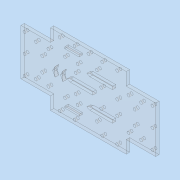
# Autodesk Inventor part: 底盘设计3.0
Saved by Autodesk Inventor 2019 (Build 230136000, 136)
## iProperties
Created: 2020-10-19
Part Number: 底盘设计3.0
Material: 聚碳酸酯，透明
Document SubType Name: Modeling
Designer: Wang Hua
Density: 1.2 g/cm^3
Appearance: 聚碳酸酯 - 透明
Author: Wang Hua
Autodesk Inventor part; units mm, degrees
ref_plane "YZ Plane" through (0, 0, 0) normal (1, 0, 0) x (0, 1, 0)
ref_plane "XZ Plane" through (0, 0, 0) normal (0, 1, 0) x (-1, 0, 0)
ref_plane "XY Plane" through (0, 0, 0) normal (0, 0, 1) x (1, 0, 0)
sketch "草图1" plane through (0, 0, 0) normal (0, 0, 1) x (1, 0, 0)
  line L0 (45, -42.5) -> (-45, -42.5)
  line L1 (-80, -27.5) -> (-80, 27.5)
  line L2 (-45, 42.5) -> (45, 42.5)
  line L3 (80, 27.5) -> (80, -27.5)
  line L4 (80, -42.5) -> (-80, 42.5) construction
  line L5 (-80, -42.5) -> (80, 42.5) construction
  line L6 (-80, -42.5) -> (-45, -42.5) construction
  line L7 (-45, -42.5) -> (-45, -27.5)
  line L8 (-45, -27.5) -> (-80, -27.5)
  line L9 (-80, -27.5) -> (-80, -42.5) construction
  line L10 (0, 0) -> (-55.8676, 0) construction
  line L11 (0, 0) -> (0, 33.8788) construction
  line L12 (-45, 42.5) -> (-45, 27.5)
  line L13 (-45, 27.5) -> (-80, 27.5)
  line L14 (45, -42.5) -> (45, -27.5)
  line L15 (45, -27.5) -> (80, -27.5)
  line L16 (45, 27.5) -> (80, 27.5)
  line L17 (45, 42.5) -> (45, 27.5)
  line L18 (-39.4263, 5.5352) -> (-42.3668, 0)
  line L19 (-30.1527, 5.5352) -> (-33.0933, 0)
  line L20 (-39.4263, -5.5352) -> (-42.3668, 0)
  line L21 (-30.1527, -5.5352) -> (-33.0933, 0)
  line L22 (-39.4263, 5.5352) -> (-40.4535, 0)
  line L23 (-30.1527, 5.5352) -> (-31.18, 0)
  line L24 (-39.4263, -5.5352) -> (-40.4535, 0)
  line L25 (-30.1527, -5.5352) -> (-31.18, 0)
  line L26 (5.2338, -1.65) -> (-21.5422, -1.65)
  line L27 (-21.5422, 1.65) -> (5.2338, 1.65)
  line L28 (5.2338, 1.65) -> (5.2338, -1.65)
  line L29 (5.2338, -1.65) -> (-21.5422, 1.65) construction
  line L30 (-21.5422, -1.65) -> (5.2338, 1.65) construction
  line L31 (-21.5422, 1.65) -> (-25.0273, 0)
  line L32 (-21.5422, -1.65) -> (-25.0273, 0)
  line L33 (-56.6923, -25.2441) -> (103.3077, 59.7559) construction
  line L34 (28.5415, 15.6059) -> (1.7655, 15.6059)
  line L35 (1.7655, 18.9059) -> (28.5415, 18.9059)
  line L36 (28.5415, 18.9059) -> (28.5415, 15.6059)
  line L37 (1.7655, 18.9059) -> (-1.7197, 17.2559)
  line L38 (1.7655, 15.6059) -> (-1.7197, 17.2559)
  line L39 (1.7655, -18.9059) -> (28.5415, -18.9059)
  line L40 (28.5415, -18.9059) -> (28.5415, -15.6059)
  line L41 (28.5415, -15.6059) -> (1.7655, -15.6059)
  line L42 (1.7655, -15.6059) -> (-1.7197, -17.2559)
  line L43 (1.7655, -18.9059) -> (-1.7197, -17.2559)
  line L44 (-27.9338, 31.5327) -> (-11.0458, 31.5327)
  line L45 (-11.0458, 31.5327) -> (-11.0458, 29.5322)
  line L46 (-11.0458, 29.5322) -> (-27.9338, 29.5322)
  line L47 (-27.9338, 29.5322) -> (-27.9338, 31.5327)
  line L48 (-27.9338, -31.5327) -> (-11.0458, -31.5327)
  line L49 (-11.0458, -31.5327) -> (-11.0458, -29.5322)
  line L50 (-11.0458, -29.5322) -> (-27.9338, -29.5322)
  line L51 (-27.9338, -29.5322) -> (-27.9338, -31.5327)
  point P0 (-62.5, 19.2523)
  point P1 (-47.5406, 19.2523)
  point P2 (-34.2099, 37.9926)
  point P3 (-16.4356, 37.9926)
  point P4 (-62.5, -19.2523)
  point P5 (-47.5406, -19.2523)
  point P6 (-34.2099, -37.9926)
  point P7 (-16.4356, -37.9926)
  point P8 (0, 37.9926)
  point P9 (62.5, 19.2523)
  point P10 (47.5406, 19.2523)
  point P11 (34.2099, 37.9926)
  point P12 (16.4356, 37.9926)
  point P13 (16.4356, -37.9926)
  point P14 (34.2099, -37.9926)
  point P15 (47.5406, -19.2523)
  point P16 (62.5, -19.2523)
  point P17 (-8.1542, 0)
  point P18 (-27.9338, 21.1189)
  point P19 (-12.8958, 21.1189)
  point P20 (-15.067, 10.9368)
  point P21 (-54.892, 8.4055)
  point P22 (-27.9338, -21.1189)
  point P23 (-12.8958, -21.1189)
  point P24 (-15.067, -10.9368)
  point P25 (-54.892, -8.4055)
  point P26 (54.892, 8.4055)
  point P27 (54.892, -8.4055)
  point P28 (15.067, 10.9368)
  point P29 (15.067, -10.9368)
  point P30 (34.2099, 8.4055)
  point P31 (34.2099, -8.4055)
  point P32 (10.0228, 26.427)
  point P33 (10.0228, -26.427)
  point P34 (-75.9408, -22.7627)
  point P35 (-75.9408, 22.7627)
  point P36 (75.9408, -22.7627)
  point P37 (75.9408, 22.7627)
  point P38 (-75.9408, 0)
  point P39 (75.9408, 0)
  dimension "d2" = 35
  dimension "d3" = 15
  dimension "d4" = 3.3
  dimension "d5" = 3.3
  dimension "d6" = 85
  dimension "d7" = 160
  constraints: 104 end point, 47 symmetric about line, 10 parallel, 9 point on line, 6 horizontal, 4 midpoint, 3 perpendicular, 1 vertical
  measures "d2" distance of L1.start L7.end
  measures "d3" distance of L0.end L7.end
  measures "d4" distance between parallel lines of L26 L27
  measures "d5" distance between parallel lines of L34 L35
  measures "d6" distance between parallel lines of L0 L2
  measures "d7" distance between parallel lines of L3 L1
extrude "拉伸1" add sketch "草图1" along normal blind 4
hole "孔1" at (-62.5, 19.2523, 0) at (-47.5406, 19.2523, 0) at (-34.2099, 37.9926, 0) at (-16.4356, 37.9926, 0) at (-16.4356, -37.9926, 0) at (-34.2099, -37.9926, 0) at (-47.5406, -19.2523, 0) at (-62.5, -19.2523, 0) at (0, 37.9926, 0) at (34.2099, 37.9926, 0) at (16.4356, 37.9926, 0) at (47.5406, 19.2523, 0) at (62.5, 19.2523, 0) at (47.5406, -19.2523, 0) at (62.5, -19.2523, 0) at (34.2099, -37.9926, 0) at (16.4356, -37.9926, 0) at (-27.9338, 21.1189, 0) at (-12.8958, 21.1189, 0) at (-15.067, 10.9368, 0) at (-54.892, 8.4055, 0) at (-54.892, -8.4055, 0) at (-15.067, -10.9368, 0) at (-12.8958, -21.1189, 0) at (-27.9338, -21.1189, 0) at (54.892, -8.4055, 0) at (54.892, 8.4055, 0) at (15.067, 10.9368, 0) at (15.067, -10.9368, 0) at (34.2099, 8.4055, 0) at (34.2099, -8.4055, 0) at (10.0228, 26.427, 0) at (10.0228, -26.427, 0) direction (0, 0, 1) diameter 3.3 end through all
hole "孔2" at (-75.9408, -22.7627, 0) at (-75.9408, 22.7627, 0) at (75.9408, -22.7627, 0) at (75.9408, 22.7627, 0) direction (0, 0, 1) diameter 3.3 end through all
hole "孔3" at (-75.9408, 0, 0) at (75.9408, 0, 0) direction (0, 0, 1) diameter 3.3 end through all
